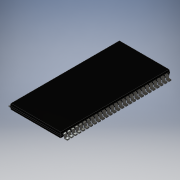
# Autodesk Inventor part: SDRAM_54SOIC
Saved by Autodesk Inventor 2016 (Build 200138000, 138)
## iProperties
Created: 2017-03-03
Part Number: SDRAM_54SOIC
Material: Generic
Document SubType Name: Modeling
Designer: jfixelle
Density: 1 g/cm^3
Appearance: Smooth - Black
Author: jfixelle
Autodesk Inventor part; units mm, degrees
ref_plane "YZ Plane" through (0, 0, 0) normal (1, 0, 0) x (0, 1, 0)
ref_plane "XZ Plane" through (0, 0, 0) normal (0, 1, 0) x (-1, 0, 0)
ref_plane "XY Plane" through (0, 0, 0) normal (0, 0, 1) x (1, 0, 0)
sketch "Sketch1" plane through (0, 0, 0) normal (0, 1, 0) x (-1, 0, 0)
  line L0 (5.145, 11.175) -> (-5.145, 11.175)
  line L1 (-5.145, 11.175) -> (-5.145, -11.175)
  line L2 (-5.145, -11.175) -> (5.145, -11.175)
  line L3 (5.145, -11.175) -> (5.145, 11.175)
  point P0 (0, 0)
  dimension "d0" = 22.35
  dimension "d1" = 11.175
  dimension "d2" = 10.29
  dimension "d3" = 5.145
  constraints: 8 end point, 2 parallel, 1 horizontal, 1 perpendicular
  measures "d0" distance of L2.end L0.start
  measures "d1" distance from line of L2 point (0, 0)
  measures "d2" distance of L1.end L2.end
  measures "d3" distance from line of point (0, 0) L3
extrude "Extrusion1" add sketch "Sketch1" along normal blind 1.1
chamfer "Chamfer1" distance 0.4 angle 10 1 edges at (0, 1.1, 11.175) measured on face at (-1.715, 0.7333, 11.175)
chamfer "Chamfer2" distance 0.4 angle 10 1 edges at (5.145, 1.1, -0.0353) measured on face at (5.145, 0.3667, 3.7015)
chamfer "Chamfer3" distance 0.4 angle 10 1 edges at (-0.0353, 1.1, -11.175) measured on face at (1.6915, 0.3667, -11.175)
chamfer "Chamfer4" distance 0.4 angle 10 1 edges at (-5.145, 1.1, 0) measured on face at (-5.145, 0.3667, -3.7015)
chamfer "Chamfer5" distance 0.4 angle 10 1 edges at (-5.145, 0, 0) measured on face at (-5.145, 0.4667, 3.725)
chamfer "Chamfer6" distance 0.4 angle 10 1 edges at (0.0353, 0, -11.175) measured on face at (-1.6915, 0.4667, -11.175)
chamfer "Chamfer7" distance 0.4 angle 10 1 edges at (0.0353, 0, 11.175) measured on face at (-1.6915, 0.4667, 11.175)
chamfer "Chamfer8" distance 0.4 angle 10 1 edges at (5.145, 0, 0) measured on face at (5.145, 0.4667, -3.7015)
sketch "Sketch2" plane through (0, 0, 0) normal (0, 0, 1) x (1, 0, 0)
  line L0 (-4.7785, 0.6446) -> (-4.7785, 0.4346)
  line L1 (-4.7785, 0.4346) -> (-5.2557, 0.4346)
  line L2 (-5.2557, 0.4346) -> (-5.385, -0.2)
  line L3 (-5.385, -0.2) -> (-5.985, -0.2)
  line L4 (-5.985, -0.2) -> (-5.985, 0.01)
  line L5 (-5.985, 0.01) -> (-5.5565, 0.01)
  line L6 (-5.5565, 0.01) -> (-5.4272, 0.6446)
  line L7 (-4.7785, 0.6446) -> (-5.4272, 0.6446)
  line L8 (-5.145, 0.4) -> (-5.145, 0.7) projected
  line L9 (5.0745, 0) -> (-5.0745, 0) projected
  line L10 (-4.8146, 0) -> (-4.6269, 0)
  point P0 (0, 0)
  dimension "d30" = 0.84
  dimension "d31" = 0.2
  dimension "d32" = 0.6
  dimension "d33" = 0.21
  dimension "d34" = 0.21
  dimension "d35" = 0.21
  constraints: 18 end point, 3 perpendicular, 2 point on line, 1 horizontal, 1 parallel
  measures "d30" distance between parallel lines of L4 L8
  measures "d31" distance between parallel lines of L3 L9
  measures "d32" distance of L2.end L3.end
  measures "d33" distance between parallel lines of L3 L5
  measures "d34" distance between parallel lines of L1 L7
  measures "d35" distance between parallel lines of L6 L2
extrude "Extrusion2" add sketch "Sketch2" along normal mid plane 0.45
pattern_linear "Rectangular Pattern1" count 27 spacing 0.8 along (0, 0, -1) of "Extrusion2" first direction both ways yes
mirror "Mirror1" about plane through (0, 0, 0) normal (1, 0, 0) of "Extrusion2", "Rectangular Pattern1"
body "Solid1"
